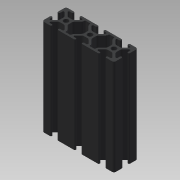
# Autodesk Inventor part: 25-2576-BLACK-FB
Saved by Autodesk Inventor 2013 (Build 170138000, 138)
## iProperties
Company: 80/20 Inc.
Created: 2014-04-23
Part Number: 25-2576-BLACK-FB
Material: Generic
Document SubType Name: Modeling
Designer: Ross Bowman
Density: 1 g/cm^3
Engineer: Ross Bowman
Catalog Web Link: 8020.net
Vendor: 80/20 Inc.
Material: 6105-T5 Aluminum
Author: Ross Bowman
Keywords: 80/20 , 8020 , T-Slot , Extrusion
Autodesk Inventor part; units mm, degrees
ref_plane "YZ Plane" through (0, 0, 0) normal (1, 0, 0) x (0, 1, 0)
ref_plane "XZ Plane" through (0, 0, 0) normal (0, 1, 0) x (-1, 0, 0)
ref_plane "XY Plane" through (0, 0, 0) normal (0, 0, 1) x (1, 0, 0)
sketch "Sketch1" plane through (0, 0, 0) normal (0, 0, 1) x (1, 0, 0)
  line L0 (4.3718, -10.36) -> (6.4282, -10.36)
  arc A0 (4.3718, -10.36) -> (4.32, -12.5) centre (4.32, -11.4294) ccw
  line L1 (4.32, -12.5) -> (20.6719, -12.5)
  arc A1 (20.6719, -12.5) -> (20.4852, -10.36) centre (20.6719, -11.4219) ccw
  line L2 (18.5718, -10.36) -> (20.4852, -10.36)
  arc A2 (17.8634, -8.6498) -> (18.5718, -10.36) centre (18.5718, -9.3582) ccw
  line L3 (17.8634, -8.6498) -> (21.1867, -5.3265)
  arc A3 (23.4235, -4.4) -> (21.1867, -5.3265) centre (23.4235, -7.5634) ccw
  line L4 (23.4235, -4.4) -> (26.5765, -4.4)
  arc A4 (28.8133, -5.3265) -> (26.5765, -4.4) centre (26.5765, -7.5634) ccw
  line L5 (28.8133, -5.3265) -> (32.1366, -8.6498)
  arc A5 (31.4282, -10.36) -> (32.1366, -8.6498) centre (31.4282, -9.3582) ccw
  line L6 (31.4282, -10.36) -> (29.5148, -10.36)
  arc A6 (29.5148, -10.36) -> (29.3281, -12.5) centre (29.3281, -11.4219) ccw
  line L7 (35.5352, -12.5) -> (29.3281, -12.5)
  arc A7 (35.5352, -12.5) -> (37.5, -10.5352) centre (35.5352, -10.5352) ccw
  line L8 (37.5, -10.5352) -> (37.5, -4.32)
  arc A8 (37.5, -4.32) -> (35.36, -4.32) centre (36.43, -4.32) ccw
  line L9 (35.36, -6.4282) -> (35.36, -4.32)
  arc A9 (33.6498, -7.1366) -> (35.36, -6.4282) centre (34.3582, -6.4282) ccw
  line L10 (33.6498, -7.1366) -> (30.3265, -3.8133)
  arc A10 (29.4, -1.5765) -> (30.3265, -3.8133) centre (32.5634, -1.5765) ccw
  line L11 (29.4, -1.5765) -> (29.4, 1.5765)
  arc A11 (30.3265, 3.8133) -> (29.4, 1.5765) centre (32.5634, 1.5765) ccw
  line L12 (30.3265, 3.8133) -> (33.6498, 7.1366)
  arc A12 (35.36, 6.4282) -> (33.6498, 7.1366) centre (34.3582, 6.4282) ccw
  line L13 (35.36, 6.4282) -> (35.36, 4.32)
  arc A13 (35.36, 4.32) -> (37.5, 4.32) centre (36.43, 4.32) ccw
  line L14 (37.5, 4.32) -> (37.5, 10.5352)
  arc A14 (37.5, 10.5352) -> (35.5352, 12.5) centre (35.5352, 10.5352) ccw
  line L15 (35.5352, 12.5) -> (29.5148, 12.5)
  arc A15 (29.5148, 12.5) -> (29.5148, 10.36) centre (29.5148, 11.43) ccw
  line L16 (29.5148, 10.36) -> (31.4282, 10.36)
  arc A16 (32.1366, 8.6498) -> (31.4282, 10.36) centre (31.4282, 9.3582) ccw
  line L17 (32.1366, 8.6498) -> (28.8133, 5.3265)
  arc A17 (26.5765, 4.4) -> (28.8133, 5.3265) centre (26.5765, 7.5634) ccw
  line L18 (26.5765, 4.4) -> (23.4235, 4.4)
  arc A18 (21.1867, 5.3265) -> (23.4235, 4.4) centre (23.4235, 7.5634) ccw
  line L19 (17.8634, 8.6498) -> (21.1867, 5.3265)
  arc A19 (18.5718, 10.36) -> (17.8634, 8.6498) centre (18.5718, 9.3582) ccw
  line L20 (18.5718, 10.36) -> (20.4852, 10.36)
  arc A20 (20.4852, 10.36) -> (20.4852, 12.5) centre (20.4852, 11.43) ccw
  line L21 (4.32, 12.5) -> (20.4852, 12.5)
  arc A21 (4.32, 12.5) -> (4.32, 10.36) centre (4.32, 11.43) ccw
  line L22 (4.32, 10.36) -> (6.4282, 10.36)
  arc A22 (7.1366, 8.6498) -> (6.4282, 10.36) centre (6.4282, 9.3582) ccw
  line L23 (7.1366, 8.6498) -> (3.8133, 5.3265)
  arc A23 (1.5765, 4.4) -> (3.8133, 5.3265) centre (1.5765, 7.5634) ccw
  line L24 (-1.5765, 4.4) -> (1.5765, 4.4)
  arc A24 (-3.8133, 5.3265) -> (-1.5765, 4.4) centre (-1.5765, 7.5634) ccw
  line L25 (-7.1366, 8.6498) -> (-3.8133, 5.3265)
  arc A25 (-6.4282, 10.36) -> (-7.1366, 8.6498) centre (-6.4282, 9.3582) ccw
  line L26 (-6.4282, 10.36) -> (-4.32, 10.36)
  arc A26 (-4.32, 10.36) -> (-4.32, 12.5) centre (-4.32, 11.43) ccw
  line L27 (-20.68, 12.5) -> (-4.32, 12.5)
  arc A27 (-20.68, 12.5) -> (-20.68, 10.36) centre (-20.68, 11.43) ccw
  line L28 (-20.68, 10.36) -> (-18.5718, 10.36)
  arc A28 (-17.8984, 8.6164) -> (-18.5718, 10.36) centre (-18.5718, 9.3582) ccw
  line L29 (-17.8984, 8.6164) -> (-21.6383, 5.2212)
  arc A29 (-23.7647, 4.4) -> (-21.6383, 5.2212) centre (-23.7647, 7.5634) ccw
  line L30 (-26.5765, 4.4) -> (-23.7647, 4.4)
  arc A30 (-28.8133, 5.3265) -> (-26.5765, 4.4) centre (-26.5765, 7.5634) ccw
  line L31 (-32.1366, 8.6498) -> (-28.8133, 5.3265)
  arc A31 (-31.4282, 10.36) -> (-32.1366, 8.6498) centre (-31.4282, 9.3582) ccw
  line L32 (-31.4282, 10.36) -> (-29.32, 10.36)
  arc A32 (-29.32, 10.36) -> (-29.32, 12.5) centre (-29.32, 11.43) ccw
  line L33 (-35.5352, 12.5) -> (-29.32, 12.5)
  arc A33 (-35.5352, 12.5) -> (-37.5, 10.5352) centre (-35.5352, 10.5352) ccw
  line L34 (-37.5, 10.5352) -> (-37.5, 4.32)
  arc A34 (-37.5, 4.32) -> (-35.36, 4.32) centre (-36.43, 4.32) ccw
  line L35 (-35.36, 4.32) -> (-35.36, 6.4282)
  arc A35 (-33.6498, 7.1366) -> (-35.36, 6.4282) centre (-34.3582, 6.4282) ccw
  line L36 (-33.6498, 7.1366) -> (-30.3265, 3.8133)
  arc A36 (-29.4, 1.5794) -> (-30.3265, 3.8133) centre (-32.5634, 1.5765) ccw
  line L37 (-29.4, 1.5794) -> (-29.4, -1.5765)
  arc A37 (-30.3265, -3.8133) -> (-29.4, -1.5765) centre (-32.5634, -1.5765) ccw
  line L38 (-30.3265, -3.8133) -> (-33.6498, -7.1366)
  arc A38 (-35.36, -6.4282) -> (-33.6498, -7.1366) centre (-34.3582, -6.4282) ccw
  line L39 (-35.36, -6.4282) -> (-35.36, -4.32)
  arc A39 (-35.36, -4.32) -> (-37.5, -4.32) centre (-36.43, -4.32) ccw
  line L40 (-37.5, -10.5352) -> (-37.5, -4.32)
  arc A40 (-37.5, -10.5352) -> (-35.5352, -12.5) centre (-35.5352, -10.5352) ccw
  line L41 (-35.5352, -12.5) -> (-29.32, -12.5)
  arc A41 (-29.32, -12.5) -> (-29.32, -10.36) centre (-29.32, -11.43) ccw
  line L42 (-31.4282, -10.36) -> (-29.32, -10.36)
  arc A42 (-32.1366, -8.6498) -> (-31.4282, -10.36) centre (-31.4282, -9.3582) ccw
  line L43 (-32.1366, -8.6498) -> (-29.1088, -5.622)
  arc A43 (-26.6112, -4.4) -> (-29.1088, -5.622) centre (-26.6112, -7.5634) ccw
  line L44 (-26.6112, -4.4) -> (-23.4235, -4.4)
  arc A44 (-21.1867, -5.3265) -> (-23.4235, -4.4) centre (-23.4235, -7.5634) ccw
  line L45 (-21.1867, -5.3265) -> (-17.8634, -8.6498)
  arc A45 (-18.5718, -10.36) -> (-17.8634, -8.6498) centre (-18.5718, -9.3582) ccw
  line L46 (-20.68, -10.36) -> (-18.5718, -10.36)
  arc A46 (-20.68, -10.36) -> (-20.68, -12.5) centre (-20.68, -11.43) ccw
  line L47 (-20.68, -12.5) -> (-4.32, -12.5)
  arc A47 (-4.32, -12.5) -> (-4.3718, -10.36) centre (-4.32, -11.4294) ccw
  line L48 (-6.4282, -10.36) -> (-4.3718, -10.36)
  arc A48 (-7.1366, -8.6498) -> (-6.4282, -10.36) centre (-6.4282, -9.3582) ccw
  line L49 (-7.1366, -8.6498) -> (-3.8133, -5.3265)
  arc A49 (-1.5765, -4.4) -> (-3.8133, -5.3265) centre (-1.5765, -7.5634) ccw
  line L50 (-1.5765, -4.4) -> (1.5765, -4.4)
  arc A50 (3.8133, -5.3265) -> (1.5765, -4.4) centre (1.5765, -7.5634) ccw
  line L51 (7.1366, -8.6498) -> (3.8133, -5.3265)
  arc A51 (6.4282, -10.36) -> (7.1366, -8.6498) centre (6.4282, -9.3582) ccw
  arc A52 (9.728, -9.6553) -> (10.4902, -10.4175) centre (10.4902, -9.6553) ccw
  line L52 (9.728, -9.6553) -> (9.728, -9.5443)
  arc A53 (9.728, -9.5443) -> (8.7995, -7.3028) centre (6.558, -9.5443) ccw
  line L53 (5.3476, -3.8509) -> (8.7995, -7.3028)
  arc A54 (4.421, -1.614) -> (5.3476, -3.8509) centre (7.5845, -1.614) ccw
  line L54 (4.421, 1.5389) -> (4.421, -1.614)
  arc A55 (5.3476, 3.7758) -> (4.421, 1.5389) centre (7.5845, 1.5389) ccw
  line L55 (8.7421, 7.1704) -> (5.3476, 3.7758)
  arc A56 (8.7421, 7.1704) -> (9.6706, 9.4119) centre (6.5006, 9.4119) ccw
  line L56 (9.6706, 9.4119) -> (9.6706, 9.5983)
  arc A57 (10.461, 10.36) -> (9.6706, 9.5983) centre (10.4328, 9.5983) ccw
  line L57 (10.461, 10.36) -> (14.6679, 10.36)
  arc A58 (15.4301, 9.5978) -> (14.6679, 10.36) centre (14.6679, 9.5978) ccw
  line L58 (15.4301, 9.5978) -> (15.4301, 9.4119)
  arc A59 (15.4301, 9.4119) -> (16.35, 7.1363) centre (18.5718, 9.3582) ccw
  line L59 (16.35, 7.1363) -> (19.6735, 3.8133)
  arc A60 (20.6, 1.5765) -> (19.6735, 3.8133) centre (17.4366, 1.5765) ccw
  line L60 (20.6, -1.5765) -> (20.6, 1.5765)
  arc A61 (19.6735, -3.8133) -> (20.6, -1.5765) centre (17.4366, -1.5765) ccw
  line L61 (16.3303, -7.1166) -> (19.6735, -3.8133)
  arc A62 (16.3303, -7.1166) -> (15.4018, -9.3582) centre (18.5718, -9.3582) ccw
  line L62 (15.4018, -9.3582) -> (15.4018, -9.6574)
  arc A63 (14.6971, -10.4175) -> (15.4018, -9.6574) centre (14.6396, -9.6574) ccw
  line L63 (10.4902, -10.4175) -> (14.6971, -10.4175)
  arc A64 (-9.6706, 9.4119) -> (-8.7421, 7.1704) centre (-6.5006, 9.4119) ccw
  line L64 (-8.7421, 7.1704) -> (-5.3476, 3.7758)
  arc A65 (-4.421, 1.5389) -> (-5.3476, 3.7758) centre (-7.5845, 1.5389) ccw
  line L65 (-4.421, 1.5389) -> (-4.421, -1.614)
  arc A66 (-5.3476, -3.8509) -> (-4.421, -1.614) centre (-7.5845, -1.614) ccw
  line L66 (-8.7995, -7.3028) -> (-5.3476, -3.8509)
  arc A67 (-8.7995, -7.3028) -> (-9.728, -9.5443) centre (-6.558, -9.5443) ccw
  line L67 (-9.728, -9.6553) -> (-9.728, -9.5443)
  arc A68 (-10.4902, -10.4175) -> (-9.728, -9.6553) centre (-10.4902, -9.6553) ccw
  line L68 (-14.6971, -10.4175) -> (-10.4902, -10.4175)
  arc A69 (-15.4018, -9.6574) -> (-14.6971, -10.4175) centre (-14.6396, -9.6574) ccw
  line L69 (-15.4018, -9.3582) -> (-15.4018, -9.6574)
  arc A70 (-15.4018, -9.3582) -> (-16.3303, -7.1166) centre (-18.5718, -9.3582) ccw
  line L70 (-16.3303, -7.1166) -> (-19.6735, -3.8133)
  arc A71 (-20.6, -1.5765) -> (-19.6735, -3.8133) centre (-17.4366, -1.5765) ccw
  line L71 (-20.6, -1.5765) -> (-20.6, 1.5765)
  arc A72 (-19.6735, 3.8133) -> (-20.6, 1.5765) centre (-17.4366, 1.5765) ccw
  line L72 (-19.6735, 3.8133) -> (-16.35, 7.1363)
  arc A73 (-16.35, 7.1363) -> (-15.4301, 9.4119) centre (-18.5718, 9.3582) ccw
  line L73 (-15.4301, 9.5978) -> (-15.4301, 9.4119)
  arc A74 (-14.6679, 10.36) -> (-15.4301, 9.5978) centre (-14.6679, 9.5978) ccw
  line L74 (-14.6679, 10.36) -> (-10.461, 10.36)
  arc A75 (-9.6706, 9.5983) -> (-10.461, 10.36) centre (-10.4328, 9.5983) ccw
  line L75 (-9.6706, 9.4119) -> (-9.6706, 9.5983)
  circle A76 centre (-25, 0) radius 2.5
  circle A77 centre (0, 0) radius 2.5
  circle A78 centre (25, 0) radius 2.5
  constraints: 152 end point, 152 point on circle, 79 centre point
extrude "Extrusion1" add sketch "Sketch1" against normal blind 100
body "Solid1"
